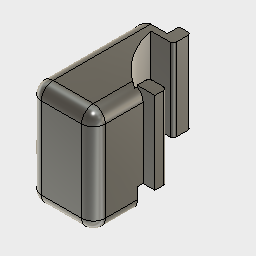
Qnap TS-210 Feet v3 (Autodesk Fusion 360 design; units mm, degrees)
Autodesk Fusion 360 part; units mm, degrees
sketch "Sketch1" plane through (0, 0, 0) normal (0, 0, 1) x (1, 0, 0) in component "Component"
  circle A0 centre (12.2295, 11.5051) radius 15
  line L0 (5.4, -9.25) -> (-5.4, -9.25)
  line L1 (-5.4, -9.25) -> (-5.4, 9.25)
  line L2 (-5.4, 9.25) -> (5.4, 9.25)
  line L3 (5.4, 9.25) -> (5.4, -9.25)
  line L4 (5.4, -9.25) -> (-5.4, 9.25) construction
  line L5 (-5.4, -9.25) -> (5.4, 9.25) construction
  line L6 (-2.6, 9.25) -> (-2.6, -9.25) construction
  line L7 (5.4, -1.85) -> (-5.4, -1.85) construction
  dimension "d1" = 30
  dimension "d2" = 18.5
  dimension "d3" = 10.8
  dimension "d4" = 2.8
  dimension "d5" = 7.4
  measures "d1" diameter of A0
  measures "d2" distance of L0.end L1.end
  measures "d3" distance of L1.end L2.end
  measures "d4" distance of L1 L6
  measures "d5" distance of L0 L7
extrude "Extrude1" add sketch "Sketch1" along normal blind 17.8 contours A0 L0 L1 L2 L3 in component "Component"
ref_plane "WorkPlane1" through (0, 0, 8.9) normal (0, 0, 1) x (1, 0, 0) in component "Component"
sketch "Sketch2" plane through (0, 0, 8.9) normal (0, 0, 1) x (1, 0, 0) in component "Component"
  line L0 (7.4, -0.85) -> (4.4, -0.85)
  line L1 (4.4, -0.85) -> (4.4, 1.15)
  line L2 (4.4, 1.15) -> (7.4, 1.15)
  line L3 (7.4, 1.15) -> (7.4, -0.85)
  line L4 (7.4, -0.85) -> (4.4, 1.15) construction
  line L5 (4.4, -0.85) -> (7.4, 1.15) construction
  line L6 (5.4, -1.85) -> (5.4, -0.85)
  arc A0 (-2.6, 9.25) -> (5.4, -1.85) centre (12.2295, 11.5051) ccw
  line L7 (4.4, -0.85) -> (4.4, -1.2894)
  line L8 (-2.6, 9.25) -> (1.4, 9.25)
  line L9 (1.4, 9.25) -> (1.4, 8.25)
  line L10 (1.4, 8.25) -> (-2.6, 8.25)
  line L11 (-2.6, 8.25) -> (-2.6, 9.25)
  line L12 (1.4, 9.25) -> (-0.6, 9.25)
  line L13 (-0.6, 9.25) -> (-0.6, 11.25)
  line L14 (-0.6, 11.25) -> (1.4, 11.25)
  line L15 (1.4, 11.25) -> (1.4, 9.25)
  point P0 (5.4, -1.85)
  point P1 (5.9, 0.15)
  dimension "d8" = 3
  dimension "d9" = 2
  dimension "d10" = 1
  dimension "d11" = 1
  dimension "d14" = 4
  dimension "d15" = 1
  dimension "d16" = 2
  dimension "d17" = 2
  measures "d8" distance of L1.end L2.end
  measures "d9" distance of L0.end L1.end
  measures "d10" distance of P0 L1
  measures "d11" distance of L0 P0
  measures "d14" distance of A0.start L8.end
  measures "d15" distance of A0.start L10.end
  measures "d16" distance of L8.end L14.end
  measures "d17" distance of L8.end L12.end
extrude "Extrude3" add sketch "Sketch2" along normal up to surface (8.9 mm away) contours A0 L8 L9 L10 L12 | L8 L12 L13 L14 L15 in component "Component"
extrude "Extrude2" add sketch "Sketch2" along normal up to surface (8.9 mm away) contours L0 L1 L2 L3 | L0 L6 A0 L7 in component "Component"
fillet "Fillet1" radius 2 9 edges at (-5.4, 0, 17.8) (-5.4, -9.25, 8.9) (0, -9.25, 17.8) (5.4, -5.05, 17.8) (5.4, -9.25, 8.9) (5.4, -5.55, 0) (0, -9.25, 0) (-5.4, 0, 0) (-5.4, 9.25, 8.9) in component "Component"
fillet "Fillet2" radius 0.5 5 edges at (4.4, 1.15, 13.35) (7.4, 1.15, 13.35) (1.4, 11.25, 13.35) (-0.6, 11.25, 13.35) (1.4, 8.25, 13.35) in component "Component"
extrude "Extrude4" add sketch "Sketch2" against normal blind 5 contours A0 L8 L9 L10 L12 | L8 L12 L13 L14 L15 in component "Component"
extrude "Extrude5" add sketch "Sketch2" against normal blind 5 contours L0 L1 L2 L3 | L0 L6 A0 L7 in component "Component"
fillet "Fillet3" radius 0.5 4 edges at (7.4, 1.15, 6.4) (4.4, 1.15, 6.4) (1.4, 11.25, 6.4) (-0.6, 11.25, 6.4) in component "Component"
fillet "Fillet4" radius 0.5 1 edges at (1.4, 8.25, 6.4) in component "Component"
component "Component" placed x (1, 0, 0) y (0, 1, 0) z (0, 0, 1) at (0, 0, 0)
